Autodesk Inventor part; units mm, degrees
(part 7 of 9)
  arc A393 (-59.0073, -75.4846) -> (-59.0867, -78.0643) centre (-58.4312, -76.7934) ccw projected
  arc A394 (-58.3073, -75.2823) -> (-59.0073, -75.4846) centre (-57.9039, -77.9913) ccw projected
  arc A395 (-58.3073, -75.2823) -> (-57.8525, -74.7461) centre (-58.3858, -74.7547) ccw projected
  arc A396 (-57.8525, -74.7461) -> (-57.8729, -73.9401) centre (-101.8395, -75.4579) ccw projected
  arc A397 (-57.8729, -73.9401) -> (-58.3543, -73.4277) centre (-58.406, -73.9585) ccw projected
  arc A398 (-59.0637, -73.2611) -> (-58.3543, -73.4277) centre (-58.0887, -70.7017) ccw projected
  arc A399 (-59.2736, -70.6887) -> (-59.0637, -73.2611) centre (-58.5546, -71.9248) ccw projected
  arc A400 (-58.6006, -70.4094) -> (-59.2736, -70.6887) centre (-57.8965, -73.0561) ccw projected
  arc A401 (-58.6006, -70.4094) -> (-58.2088, -69.8256) centre (-58.7378, -69.8939) ccw projected
  arc A402 (-58.2088, -69.8256) -> (-58.3193, -69.027) centre (-101.8395, -75.4579) ccw projected
  arc A403 (-58.3193, -69.027) -> (-58.855, -68.5716) centre (-58.847, -69.105) ccw projected
  arc A404 (-59.5786, -68.4856) -> (-58.855, -68.5716) centre (-58.8963, -65.8331) ccw projected
  arc A405 (-60.0753, -65.9528) -> (-59.5786, -68.4856) centre (-59.2223, -67.1006) ccw projected
  arc A406 (-59.4378, -65.5999) -> (-60.0753, -65.9528) centre (-58.4417, -68.1512) ccw projected
  arc A407 (-59.4378, -65.5999) -> (-59.1137, -64.9759) centre (-59.6318, -65.103) ccw projected
  arc A408 (-59.1137, -64.9759) -> (-59.313, -64.1947) centre (-101.8395, -75.4579) ccw projected
  arc A409 (-59.313, -64.1947) -> (-59.8963, -63.8022) centre (-59.8286, -64.3313) ccw projected
  arc A410 (-60.625, -63.7977) -> (-59.8963, -63.8022) centre (-60.2439, -61.0855) ccw projected
  arc A411 (-61.4021, -61.3365) -> (-60.625, -63.7977) centre (-60.426, -62.3816) ccw projected
  arc A412 (-60.8081, -60.9144) -> (-61.4021, -61.3365) centre (-59.5327, -63.3381) ccw projected
  arc A413 (-60.8081, -60.9144) -> (-60.556, -60.2581) centre (-61.0566, -60.4424) ccw projected
  arc A414 (-60.556, -60.2581) -> (-60.8415, -59.5041) centre (-101.8395, -75.4579) ccw projected
  arc A415 (-60.8415, -59.5041) -> (-61.4651, -59.1793) centre (-61.3386, -59.6975) ccw projected
  arc A416 (-62.1896, -59.2564) -> (-61.4651, -59.1793) centre (-62.1147, -56.5186) ccw projected
  arc A417 (-63.2375, -56.8977) -> (-62.1896, -59.2564) centre (-62.1505, -57.827) ccw projected
  arc A418 (-62.6945, -56.4118) -> (-63.2375, -56.8977) centre (-61.1557, -58.6774) ccw projected
  arc A419 (-62.6945, -56.4118) -> (-62.5174, -55.7313) centre (-62.9942, -55.9705) ccw projected
  arc A420 (-62.5174, -55.7313) -> (-62.8855, -55.0141) centre (-101.8395, -75.4579) ccw projected
  arc A421 (-62.8855, -55.0141) -> (-63.5416, -54.7612) centre (-63.3578, -55.2619) ccw projected
  arc A422 (-64.253, -54.9189) -> (-63.5416, -54.7612) centre (-64.485, -52.19) ccw projected
  arc A423 (-65.5583, -52.6924) -> (-64.253, -54.9189) centre (-64.3741, -53.4941) ccw projected
  arc A424 (-65.0731, -52.1487) -> (-65.5583, -52.6924) centre (-63.2903, -54.2278) ccw projected
  arc A425 (-65.0731, -52.1487) -> (-64.9734, -51.4527) centre (-65.4203, -51.7438) ccw projected
  arc A426 (-64.9734, -51.4527) -> (-65.4195, -50.7811) centre (-101.8395, -75.4579) ccw projected
  arc A427 (-65.4195, -50.7811) -> (-66.0997, -50.6033) centre (-65.861, -51.0803) ccw projected
  arc A428 (-66.7889, -50.8397) -> (-66.0997, -50.6033) centre (-67.3251, -48.1539) ccw projected
  arc A429 (-68.3353, -48.7733) -> (-66.7889, -50.8397) centre (-67.0689, -49.4374) ccw projected
  arc A430 (-67.9141, -48.1787) -> (-68.3353, -48.7733) centre (-65.9097, -50.0451) ccw projected
  arc A431 (-67.9141, -48.1787) -> (-67.8929, -47.4759) centre (-68.3045, -47.8152) ccw projected
  arc A432 (-67.8929, -47.4759) -> (-68.4114, -46.8585) centre (-101.8395, -75.4579) ccw projected
  arc A433 (-68.4114, -46.8585) -> (-69.1073, -46.758) centre (-68.8167, -47.2053) ccw projected
  arc A434 (-69.7657, -47.0701) -> (-69.1073, -46.758) centre (-70.5992, -44.4612) ccw projected
  arc A435 (-71.5337, -45.1898) -> (-69.7657, -47.0701) centre (-70.2009, -45.7079) ccw projected
  arc A436 (-71.1817, -44.5518) -> (-71.5337, -45.1898) centre (-68.981, -46.1821) ccw projected
  arc A437 (-71.1817, -44.5518) -> (-71.2393, -43.8511) centre (-71.6104, -44.2343) ccw projected
  arc A438 (-71.2393, -43.8511) -> (-71.8237, -43.2956) centre (-101.8395, -75.4579) ccw projected
  arc A439 (-71.8237, -43.2956) -> (-72.5264, -43.2736) centre (-72.1876, -43.6856) ccw projected
  arc A440 (-73.1458, -43.6575) -> (-72.5264, -43.2736) centre (-74.2661, -41.1583) ccw projected
  arc A441 (-75.1132, -41.9869) -> (-73.1458, -43.6575) centre (-73.7308, -42.3525) ccw projected
  arc A442 (-74.8349, -41.3135) -> (-75.1132, -41.9869) centre (-72.4654, -42.6872) ccw projected
  arc A443 (-74.8349, -41.3135) -> (-74.9706, -40.6237) centre (-75.2964, -41.046) ccw projected
  arc A444 (-74.9706, -40.6237) -> (-75.6135, -40.1371) centre (-101.8395, -75.4579) ccw projected
  arc A445 (-75.6135, -40.1371) -> (-76.3143, -40.1939) centre (-75.9315, -40.5654) ccw projected
  arc A446 (-76.8867, -40.6447) -> (-76.3143, -40.1939) centre (-78.2798, -38.2867) ccw projected
  arc A447 (-79.0289, -39.205) -> (-76.8867, -40.6447) centre (-77.6141, -39.4135) ccw projected
  arc A448 (-78.8277, -38.5047) -> (-79.0289, -39.205) centre (-76.3193, -39.6044) ccw projected
  arc A449 (-78.8277, -38.5047) -> (-79.0397, -37.8343) centre (-79.3162, -38.2905) ccw projected
  arc A450 (-79.0397, -37.8343) -> (-79.7331, -37.4228) centre (-101.8395, -75.4579) ccw projected
  arc A451 (-79.7331, -37.4228) -> (-80.4231, -37.5577) centre (-80.0011, -37.884) ccw projected
  arc A452 (-80.9415, -38.0698) -> (-80.4231, -37.5577) centre (-82.5898, -35.8826) ccw projected
  arc A453 (-83.2313, -36.879) -> (-80.9415, -38.0698) centre (-81.8021, -36.9278) ccw projected
  arc A454 (-83.1098, -36.1605) -> (-83.2313, -36.879) centre (-80.4941, -36.9724) ccw projected
  arc A455 (-83.1098, -36.1605) -> (-83.3956, -35.5181) centre (-83.6192, -36.0024) ccw projected
  arc A456 (-83.3956, -35.5181) -> (-84.1306, -35.1868) centre (-101.8395, -75.4579) ccw projected
  line L37 (-121.8728, 32.134) -> (-90.1228, 6.734)
  line L38 (-121.8728, 6.734) -> (-90.1228, 32.134)
  circle A457 centre (-171.542, -73.2557) radius 14.2748
  circle A458 centre (-105.9978, 19.434) radius 21.4859
  circle A459 centre (-171.542, -73.2557) radius 14.3243
  line L39 (-160.3914, -82.2474) -> (-89.2724, 5.9468)
  line L40 (-124.2883, 30.7078) -> (-183.736, -65.7396)
  line L41 (-193.767, -95.4807) -> (-149.317, -95.4807)
  line L42 (-149.317, -95.4807) -> (-149.317, -51.0307)
  line L43 (-149.317, -51.0307) -> (-193.767, -51.0307)
  line L44 (-193.767, -51.0307) -> (-193.767, -95.4807)
  line L45 (-193.767, -95.4807) -> (-149.317, -51.0307) construction
  line L46 (-149.317, -95.4807) -> (-193.767, -51.0307) construction
  circle A460 centre (-171.542, -73.2557) radius 31.4309
  arc A461 (-181.9312, -110.8876) -> (-185.6678, -111.3086) centre (-183.1204, -117.1252) ccw projected
  arc A462 (-174.8852, -173.4224) -> (-181.9312, -110.8876) centre (-180.2765, -142.3655) ccw projected
  arc A463 (-178.6218, -173.8435) -> (-174.8852, -173.4224) centre (-177.4326, -167.6058) ccw projected
  arc A464 (-185.6678, -111.3086) -> (-178.6218, -173.8435) centre (-180.2765, -142.3655) ccw projected
  arc A465 (-181.7907, -98.8592) -> (-182.3406, -98.4212) centre (-182.3156, -98.954) ccw projected
  arc A466 (-182.3406, -98.4212) -> (-183.1456, -98.4664) centre (-180.2765, -142.3655) ccw projected
  arc A467 (-183.1456, -98.4664) -> (-183.643, -98.9632) centre (-183.1108, -98.9986) ccw projected
  arc A468 (-183.7876, -99.6774) -> (-183.643, -98.9632) centre (-186.3758, -98.7816) ccw projected
  arc A469 (-186.3524, -99.9664) -> (-183.7876, -99.6774) centre (-185.139, -99.2097) ccw projected
  arc A470 (-186.6523, -99.3023) -> (-186.3524, -99.9664) centre (-184.0285, -98.5171) ccw projected
  arc A471 (-186.6523, -99.3023) -> (-187.2478, -98.9286) centre (-187.1633, -99.4552) ccw projected
  arc A472 (-187.2478, -98.9286) -> (-188.0427, -99.0636) centre (-180.2765, -142.3655) ccw projected
  arc A473 (-188.0427, -99.0636) -> (-188.4814, -99.6131) centre (-187.9485, -99.5887) ccw projected
  arc A474 (-188.5451, -100.3389) -> (-188.4814, -99.6131) centre (-191.2173, -99.7385) ccw projected
  arc A475 (-191.0614, -100.9133) -> (-188.5451, -100.3389) centre (-189.9403, -100.0254) ccw projected
  arc A476 (-191.4338, -100.2869) -> (-191.0614, -100.9133) centre (-188.9143, -99.2129) ccw projected
  arc A477 (-191.4338, -100.2869) -> (-192.0674, -99.9822) centre (-191.9244, -100.4961) ccw projected
  arc A478 (-192.0674, -99.9822) -> (-192.8421, -100.2054) centre (-180.2765, -142.3655) ccw projected
  arc A479 (-192.8421, -100.2054) -> (-193.2165, -100.8006) centre (-192.6898, -100.7166) ccw projected
  arc A480 (-193.1986, -101.529) -> (-193.2165, -100.8006) centre (-195.9212, -101.2315) ccw projected
  arc A481 (-195.6348, -102.3814) -> (-193.1986, -101.529) centre (-194.6202, -101.3737) ccw projected
  arc A482 (-196.0749, -101.8007) -> (-195.6348, -102.3814) centre (-193.6916, -100.4513) ccw projected
  arc A483 (-196.0749, -101.8007) -> (-196.7387, -101.5689) centre (-196.5391, -102.0636) ccw projected
  arc A484 (-196.7387, -101.5689) -> (-197.4835, -101.8774) centre (-180.2765, -142.3655) ccw projected
  arc A485 (-197.4835, -101.8774) -> (-197.789, -102.5107) centre (-197.2749, -102.3683) ccw projected
  arc A486 (-197.6896, -103.2326) -> (-197.789, -102.5107) centre (-200.4284, -103.2418) ccw projected
  arc A487 (-200.015, -104.3524) -> (-197.6896, -103.2326) centre (-199.1196, -103.2374) ccw projected
  arc A488 (-200.5174, -103.8247) -> (-200.015, -104.3524) centre (-198.3001, -102.2169) ccw projected
  arc A489 (-200.5174, -103.8247) -> (-201.2029, -103.6686) centre (-200.9492, -104.1378) ccw projected
  arc A490 (-201.2029, -103.6686) -> (-201.9086, -104.0586) centre (-180.2765, -142.3655) ccw projected
  arc A491 (-201.9086, -104.0586) -> (-202.1412, -104.7221) centre (-201.6463, -104.5231) ccw projected
  arc A492 (-201.9616, -105.4283) -> (-202.1412, -104.7221) centre (-204.6822, -105.7441) ccw projected
  arc A493 (-204.147, -106.8014) -> (-201.9616, -105.4283) centre (-203.3821, -105.5932) ccw projected
  arc A494 (-204.7053, -106.3333) -> (-204.147, -106.8014) centre (-202.682, -104.4874) ccw projected
  arc A495 (-204.7053, -106.3333) -> (-205.404, -106.2549) centre (-205.0994, -106.6928) ccw projected
  arc A496 (-205.404, -106.2549) -> (-206.0616, -106.7215) centre (-180.2765, -142.3655) ccw projected
  arc A497 (-206.0616, -106.7215) -> (-206.2184, -107.4069) centre (-205.7489, -107.1537) ccw projected
  arc A498 (-205.9609, -108.0885) -> (-206.2184, -107.4069) centre (-208.629, -108.707) ccw projected
  arc A499 (-207.9788, -109.6977) -> (-205.9609, -108.0885) centre (-207.354, -108.4114) ccw projected
  arc A500 (-208.5861, -109.295) -> (-207.9788, -109.6977) centre (-206.7821, -107.2342) ccw projected
  arc A501 (-208.5861, -109.295) -> (-209.2891, -109.2954) centre (-208.9374, -109.6964) ccw projected
  arc A502 (-209.2891, -109.2954) -> (-209.8903, -109.8326) centre (-180.2765, -142.3655) ccw projected
  arc A503 (-209.8903, -109.8326) -> (-209.9694, -110.5312) centre (-209.5312, -110.2271) ccw projected
  arc A504 (-209.6372, -111.1798) -> (-209.9694, -110.5312) centre (-212.2193, -112.0931) ccw projected
  arc A505 (-211.4623, -113.0048) -> (-209.6372, -111.1798) centre (-210.9854, -111.6566) ccw projected
  arc A506 (-212.1108, -112.6726) -> (-211.4623, -113.0048) centre (-210.5489, -110.4227) ccw projected
  arc A507 (-212.1108, -112.6726) -> (-212.8094, -112.7517) centre (-212.4149, -113.1108) ccw projected
  arc A508 (-212.8094, -112.7517) -> (-213.3466, -113.3529) centre (-180.2765, -142.3655) ccw projected
  arc A509 (-213.3466, -113.3529) -> (-213.347, -114.056) centre (-212.9457, -113.7046) ccw projected
  arc A510 (-212.9443, -114.6632) -> (-213.347, -114.056) centre (-215.4079, -115.8599) ccw projected
  arc A511 (-214.5535, -116.6811) -> (-212.9443, -114.6632) centre (-214.2306, -115.288) ccw projected
  arc A512 (-215.2352, -116.4236) -> (-214.5535, -116.6811) centre (-213.9351, -114.013) ccw projected
  arc A513 (-215.2352, -116.4236) -> (-215.9205, -116.5804) centre (-215.4884, -116.8931) ccw projected
  arc A514 (-215.9205, -116.5804) -> (-216.3871, -117.238) centre (-180.2765, -142.3655) ccw projected
  arc A515 (-216.3871, -117.238) -> (-216.3087, -117.9367) centre (-215.9492, -117.5426) ccw projected
  arc A516 (-215.8406, -118.495) -> (-216.3087, -117.9367) centre (-218.1547, -119.96) ccw projected
  arc A517 (-217.2137, -120.6804) -> (-215.8406, -118.495) centre (-217.0488, -119.2599) ccw projected
  arc A518 (-217.9199, -120.5008) -> (-217.2137, -120.6804) centre (-216.8979, -117.9599) ccw projected
  arc A519 (-217.9199, -120.5008) -> (-218.5834, -120.7334) centre (-218.119, -120.9957) ccw projected
  arc A520 (-218.5834, -120.7334) -> (-218.9734, -121.4391) centre (-180.2765, -142.3655) ccw projected
  arc A521 (-218.9734, -121.4391) -> (-218.8173, -122.1246) centre (-218.5042, -121.6928) ccw projected
  arc A522 (-218.2896, -122.627) -> (-218.8173, -122.1246) centre (-220.4251, -124.3419) ccw projected
  arc A523 (-219.4094, -124.9524) -> (-218.2896, -122.627) centre (-219.4046, -123.5224) ccw projected
  arc A524 (-220.1313, -124.8531) -> (-219.4094, -124.9524) centre (-219.4002, -122.2136) ccw projected
  arc A525 (-220.1313, -124.8531) -> (-220.7646, -125.1585) centre (-220.2737, -125.3671) ccw projected
  arc A526 (-220.7646, -125.1585) -> (-221.0731, -125.9033) centre (-180.2765, -142.3655) ccw projected
  arc A527 (-221.0731, -125.9033) -> (-220.8413, -126.5671) centre (-220.5785, -126.1029) ccw projected
  arc A528 (-220.2606, -127.0073) -> (-220.8413, -126.5671) centre (-222.1907, -128.9504) ccw projected
  arc A529 (-221.113, -129.4434) -> (-220.2606, -127.0073) centre (-221.2683, -128.0218) ccw projected
  arc A530 (-221.8415, -129.4255) -> (-221.113, -129.4434) centre (-221.4105, -126.7208) ccw projected
  arc A531 (-221.8415, -129.4255) -> (-222.4366, -129.7999) centre (-221.9254, -129.9522) ccw projected
  arc A532 (-222.4366, -129.7999) -> (-222.6598, -130.5746) centre (-180.2765, -142.3655) ccw projected
  arc A533 (-222.6598, -130.5746) -> (-222.3551, -131.2083) centre (-222.1459, -130.7176) ccw projected
  arc A534 (-221.7287, -131.5806) -> (-222.3551, -131.2083) centre (-223.4291, -133.7277) ccw projected
  arc A535 (-222.3031, -134.0969) -> (-221.7287, -131.5806) centre (-222.6166, -132.7017) ccw projected
  arc A536 (-223.0289, -134.1607) -> (-222.3031, -134.0969) centre (-222.9035, -131.4247) ccw projected
  arc A537 (-223.0289, -134.1607) -> (-223.5784, -134.5993) centre (-223.0534, -134.6935) ccw projected
  arc A538 (-223.5784, -134.5993) -> (-223.7134, -135.3942) centre (-180.2765, -142.3655) ccw projected
  arc A539 (-223.7134, -135.3942) -> (-223.3397, -135.9897) centre (-223.1868, -135.4787) ccw projected
  arc A540 (-222.6756, -136.2896) -> (-223.3397, -135.9897) centre (-224.1249, -138.6136) ccw projected
  arc A541 (-222.9646, -138.8544) -> (-222.6756, -136.2896) centre (-223.4324, -137.503) ccw projected
  arc A542 (-223.6788, -138.999) -> (-222.9646, -138.8544) centre (-223.8604, -136.2662) ccw projected
  arc A543 (-223.6788, -138.999) -> (-224.1756, -139.4964) centre (-223.6434, -139.5312) ccw projected
  arc A544 (-224.1756, -139.4964) -> (-224.2209, -140.3014) centre (-180.2765, -142.3655) ccw projected
  arc A545 (-224.2209, -140.3014) -> (-223.7828, -140.8513) centre (-223.688, -140.3264) ccw projected
  arc A546 (-223.0893, -141.075) -> (-223.7828, -140.8513) centre (-224.2693, -143.5466) ccw projected
  arc A547 (-223.0893, -143.656) -> (-223.0893, -141.075) centre (-223.7054, -142.3655) ccw projected
  arc A548 (-223.7828, -143.8797) -> (-223.0893, -143.656) centre (-224.2693, -141.1844) ccw projected
  arc A549 (-223.7828, -143.8797) -> (-224.2209, -144.4296) centre (-223.688, -144.4046) ccw projected
  arc A550 (-224.2209, -144.4296) -> (-224.1756, -145.2346) centre (-180.2765, -142.3655) ccw projected
  arc A551 (-224.1756, -145.2346) -> (-223.6788, -145.732) centre (-223.6434, -145.1998) ccw projected
  arc A552 (-222.9646, -145.8766) -> (-223.6788, -145.732) centre (-223.8604, -148.4648) ccw projected
  arc A553 (-222.6756, -148.4414) -> (-222.9646, -145.8766) centre (-223.4324, -147.228) ccw projected
  arc A554 (-223.3397, -148.7413) -> (-222.6756, -148.4414) centre (-224.1249, -146.1175) ccw projected
  arc A555 (-223.3397, -148.7413) -> (-223.7134, -149.3368) centre (-223.1868, -149.2523) ccw projected
  arc A556 (-223.7134, -149.3368) -> (-223.5784, -150.1317) centre (-180.2765, -142.3655) ccw projected
  arc A557 (-223.5784, -150.1317) -> (-223.0289, -150.5704) centre (-223.0534, -150.0375) ccw projected
  arc A558 (-222.3031, -150.6341) -> (-223.0289, -150.5704) centre (-222.9035, -153.3063) ccw projected
  arc A559 (-221.7287, -153.1504) -> (-222.3031, -150.6341) centre (-222.6166, -152.0294) ccw projected
  arc A560 (-222.3551, -153.5228) -> (-221.7287, -153.1504) centre (-223.4291, -151.0033) ccw projected
  arc A561 (-222.3551, -153.5228) -> (-222.6598, -154.1564) centre (-222.1459, -154.0134) ccw projected
  arc A562 (-222.6598, -154.1564) -> (-222.4366, -154.9311) centre (-180.2765, -142.3655) ccw projected
  arc A563 (-222.4366, -154.9311) -> (-221.8415, -155.3055) centre (-221.9254, -154.7788) ccw projected
  arc A564 (-221.113, -155.2876) -> (-221.8415, -155.3055) centre (-221.4105, -158.0102) ccw projected
  arc A565 (-220.2606, -157.7238) -> (-221.113, -155.2876) centre (-221.2683, -156.7092) ccw projected
  arc A566 (-220.8413, -158.1639) -> (-220.2606, -157.7238) centre (-222.1907, -155.7806) ccw projected
  arc A567 (-220.8413, -158.1639) -> (-221.0731, -158.8277) centre (-220.5785, -158.6281) ccw projected
  arc A568 (-221.0731, -158.8277) -> (-220.7646, -159.5726) centre (-180.2765, -142.3655) ccw projected
  arc A569 (-220.7646, -159.5726) -> (-220.1313, -159.878) centre (-220.2737, -159.3639) ccw projected
  arc A570 (-219.4094, -159.7786) -> (-220.1313, -159.878) centre (-219.4002, -162.5174) ccw projected
  arc A571 (-218.2896, -162.104) -> (-219.4094, -159.7786) centre (-219.4046, -161.2086) ccw projected
  arc A572 (-218.8173, -162.6064) -> (-218.2896, -162.104) centre (-220.4251, -160.3891) ccw projected
  arc A573 (-218.8173, -162.6064) -> (-218.9734, -163.2919) centre (-218.5042, -163.0382) ccw projected
  arc A574 (-218.9734, -163.2919) -> (-218.5834, -163.9976) centre (-180.2765, -142.3655) ccw projected
  arc A575 (-218.5834, -163.9976) -> (-217.9199, -164.2302) centre (-218.119, -163.7353) ccw projected
  arc A576 (-217.2137, -164.0506) -> (-217.9199, -164.2302) centre (-216.8979, -166.7712) ccw projected
  arc A577 (-215.8406, -166.236) -> (-217.2137, -164.0506) centre (-217.0488, -165.4711) ccw projected
  arc A578 (-216.3087, -166.7943) -> (-215.8406, -166.236) centre (-218.1547, -164.771) ccw projected
  arc A579 (-216.3087, -166.7943) -> (-216.3871, -167.493) centre (-215.9492, -167.1884) ccw projected
  arc A580 (-216.3871, -167.493) -> (-215.9205, -168.1506) centre (-180.2765, -142.3655) ccw projected
  arc A581 (-215.9205, -168.1506) -> (-215.2352, -168.3074) centre (-215.4884, -167.8379) ccw projected
  arc A582 (-214.5535, -168.0499) -> (-215.2352, -168.3074) centre (-213.9351, -170.718) ccw projected
  arc A583 (-212.9443, -170.0678) -> (-214.5535, -168.0499) centre (-214.2306, -169.443) ccw projected
  arc A584 (-213.347, -170.6751) -> (-212.9443, -170.0678) centre (-215.4079, -168.8712) ccw projected
  arc A585 (-213.347, -170.6751) -> (-213.3466, -171.3781) centre (-212.9457, -171.0264) ccw projected
  arc A586 (-213.3466, -171.3781) -> (-212.8094, -171.9793) centre (-180.2765, -142.3655) ccw projected
  arc A587 (-212.8094, -171.9793) -> (-212.1108, -172.0584) centre (-212.4149, -171.6203) ccw projected
  arc A588 (-211.4623, -171.7262) -> (-212.1108, -172.0584) centre (-210.5489, -174.3083) ccw projected
  arc A589 (-209.6372, -173.5513) -> (-211.4623, -171.7262) centre (-210.9854, -173.0744) ccw projected
  arc A590 (-209.9694, -174.1998) -> (-209.6372, -173.5513) centre (-212.2193, -172.638) ccw projected
  arc A591 (-209.9694, -174.1998) -> (-209.8903, -174.8984) centre (-209.5312, -174.504) ccw projected
  arc A592 (-209.8903, -174.8984) -> (-209.2891, -175.4356) centre (-180.2765, -142.3655) ccw projected
  arc A593 (-209.2891, -175.4356) -> (-208.5861, -175.436) centre (-208.9374, -175.0347) ccw projected
  arc A594 (-207.9788, -175.0333) -> (-208.5861, -175.436) centre (-206.7821, -177.4969) ccw projected
  arc A595 (-205.9609, -176.6425) -> (-207.9788, -175.0333) centre (-207.354, -176.3196) ccw projected
  arc A596 (-206.2184, -177.3242) -> (-205.9609, -176.6425) centre (-208.629, -176.0241) ccw projected
  arc A597 (-206.2184, -177.3242) -> (-206.0616, -178.0095) centre (-205.7489, -177.5774) ccw projected
  arc A598 (-206.0616, -178.0095) -> (-205.404, -178.4761) centre (-180.2765, -142.3655) ccw projected
  arc A599 (-205.404, -178.4761) -> (-204.7053, -178.3978) centre (-205.0994, -178.0383) ccw projected
  arc A600 (-204.147, -177.9296) -> (-204.7053, -178.3978) centre (-202.682, -180.2437) ccw projected
  arc A601 (-201.9616, -179.3027) -> (-204.147, -177.9296) centre (-203.3821, -179.1378) ccw projected
  arc A602 (-202.1412, -180.0089) -> (-201.9616, -179.3027) centre (-204.6822, -178.9869) ccw projected
  arc A603 (-202.1412, -180.0089) -> (-201.9086, -180.6724) centre (-201.6463, -180.208) ccw projected
  arc A604 (-201.9086, -180.6724) -> (-201.2029, -181.0624) centre (-180.2765, -142.3655) ccw projected
  arc A605 (-201.2029, -181.0624) -> (-200.5174, -180.9064) centre (-200.9492, -180.5932) ccw projected
  arc A606 (-200.015, -180.3786) -> (-200.5174, -180.9064) centre (-198.3001, -182.5141) ccw projected
  arc A607 (-197.6896, -181.4984) -> (-200.015, -180.3786) centre (-199.1196, -181.4936) ccw projected
  arc A608 (-197.789, -182.2203) -> (-197.6896, -181.4984) centre (-200.4284, -181.4892) ccw projected
  arc A609 (-197.789, -182.2203) -> (-197.4835, -182.8536) centre (-197.2749, -182.3627) ccw projected
  arc A610 (-197.4835, -182.8536) -> (-196.7387, -183.1621) centre (-180.2765, -142.3655) ccw projected
  arc A611 (-196.7387, -183.1621) -> (-196.0749, -182.9303) centre (-196.5391, -182.6675) ccw projected
  arc A612 (-195.6348, -182.3496) -> (-196.0749, -182.9303) centre (-193.6916, -184.2797) ccw projected
  arc A613 (-193.1986, -183.202) -> (-195.6348, -182.3496) centre (-194.6202, -183.3573) ccw projected
  arc A614 (-193.2165, -183.9305) -> (-193.1986, -183.202) centre (-195.9212, -183.4995) ccw projected
  arc A615 (-193.2165, -183.9305) -> (-192.8421, -184.5256) centre (-192.6898, -184.0144) ccw projected
  arc A616 (-192.8421, -184.5256) -> (-192.0674, -184.7488) centre (-180.2765, -142.3655) ccw projected
  arc A617 (-192.0674, -184.7488) -> (-191.4338, -184.4441) centre (-191.9244, -184.2349) ccw projected
  arc A618 (-191.0614, -183.8178) -> (-191.4338, -184.4441) centre (-188.9143, -185.5181) ccw projected
  arc A619 (-188.5451, -184.3921) -> (-191.0614, -183.8178) centre (-189.9403, -184.7056) ccw projected
  arc A620 (-188.4814, -185.1179) -> (-188.5451, -184.3921) centre (-191.2173, -184.9925) ccw projected
  arc A621 (-188.4814, -185.1179) -> (-188.0427, -185.6674) centre (-187.9485, -185.1424) ccw projected
  arc A622 (-188.0427, -185.6674) -> (-187.2478, -185.8024) centre (-180.2765, -142.3655) ccw projected
  arc A623 (-187.2478, -185.8024) -> (-186.6523, -185.4287) centre (-187.1633, -185.2758) ccw projected
  arc A624 (-186.3524, -184.7646) -> (-186.6523, -185.4287) centre (-184.0285, -186.2139) ccw projected
  arc A625 (-183.7876, -185.0536) -> (-186.3524, -184.7646) centre (-185.139, -185.5214) ccw projected
  arc A626 (-183.643, -185.7678) -> (-183.7876, -185.0536) centre (-186.3758, -185.9495) ccw projected
  arc A627 (-183.643, -185.7678) -> (-183.1456, -186.2647) centre (-183.1108, -185.7324) ccw projected
  arc A628 (-183.1456, -186.2647) -> (-182.3406, -186.3099) centre (-180.2765, -142.3655) ccw projected
  arc A629 (-182.3406, -186.3099) -> (-181.7907, -185.8718) centre (-182.3156, -185.777) ccw projected
  arc A630 (-181.567, -185.1783) -> (-181.7907, -185.8718) centre (-179.0954, -186.3583) ccw projected
  arc A631 (-178.986, -185.1783) -> (-181.567, -185.1783) centre (-180.2765, -185.7944) ccw projected
  arc A632 (-178.7623, -185.8718) -> (-178.986, -185.1783) centre (-181.4576, -186.3583) ccw projected
  arc A633 (-178.7623, -185.8718) -> (-178.2124, -186.3099) centre (-178.2374, -185.777) ccw projected
  arc A634 (-178.2124, -186.3099) -> (-177.4074, -186.2647) centre (-180.2765, -142.3655) ccw projected
  arc A635 (-177.4074, -186.2647) -> (-176.91, -185.7678) centre (-177.4422, -185.7324) ccw projected
  arc A636 (-176.7654, -185.0536) -> (-176.91, -185.7678) centre (-174.1772, -185.9495) ccw projected
  arc A637 (-174.2006, -184.7646) -> (-176.7654, -185.0536) centre (-175.414, -185.5214) ccw projected
  arc A638 (-173.9007, -185.4287) -> (-174.2006, -184.7646) centre (-176.5245, -186.2139) ccw projected
  arc A639 (-173.9007, -185.4287) -> (-173.3052, -185.8024) centre (-173.3897, -185.2758) ccw projected
  arc A640 (-173.3052, -185.8024) -> (-172.5103, -185.6674) centre (-180.2765, -142.3655) ccw projected
  arc A641 (-172.5103, -185.6674) -> (-172.0716, -185.1179) centre (-172.6045, -185.1424) ccw projected
  arc A642 (-172.0079, -184.3921) -> (-172.0716, -185.1179) centre (-169.3357, -184.9925) ccw projected
  arc A643 (-169.4916, -183.8178) -> (-172.0079, -184.3921) centre (-170.6127, -184.7056) ccw projected
  arc A644 (-169.1192, -184.4441) -> (-169.4916, -183.8178) centre (-171.6387, -185.5181) ccw projected
  arc A645 (-169.1192, -184.4441) -> (-168.4856, -184.7488) centre (-168.6286, -184.2349) ccw projected
  arc A646 (-168.4856, -184.7488) -> (-167.7109, -184.5256) centre (-180.2765, -142.3655) ccw projected
  arc A647 (-167.7109, -184.5256) -> (-167.3365, -183.9305) centre (-167.8632, -184.0144) ccw projected
  arc A648 (-167.3544, -183.202) -> (-167.3365, -183.9305) centre (-164.6318, -183.4995) ccw projected
  arc A649 (-164.9183, -182.3496) -> (-167.3544, -183.202) centre (-165.9328, -183.3573) ccw projected
  arc A650 (-164.4781, -182.9303) -> (-164.9183, -182.3496) centre (-166.8614, -184.2797) ccw projected
  arc A651 (-164.4781, -182.9303) -> (-163.8143, -183.1621) centre (-164.0139, -182.6675) ccw projected
  arc A652 (-163.8143, -183.1621) -> (-163.0695, -182.8536) centre (-180.2765, -142.3655) ccw projected
  arc A653 (-163.0695, -182.8536) -> (-162.764, -182.2203) centre (-163.2781, -182.3627) ccw projected
  arc A654 (-162.8634, -181.4984) -> (-162.764, -182.2203) centre (-160.1246, -181.4892) ccw projected
  arc A655 (-160.538, -180.3786) -> (-162.8634, -181.4984) centre (-161.4334, -181.4936) ccw projected
  arc A656 (-160.0356, -180.9064) -> (-160.538, -180.3786) centre (-162.2529, -182.5141) ccw projected
  arc A657 (-160.0356, -180.9064) -> (-159.3501, -181.0624) centre (-159.6038, -180.5932) ccw projected
  arc A658 (-159.3501, -181.0624) -> (-158.6444, -180.6724) centre (-180.2765, -142.3655) ccw projected
  arc A659 (-158.6444, -180.6724) -> (-158.4118, -180.0089) centre (-158.9067, -180.208) ccw projected
  arc A660 (-158.5914, -179.3027) -> (-158.4118, -180.0089) centre (-155.8709, -178.9869) ccw projected
  arc A661 (-156.406, -177.9296) -> (-158.5914, -179.3027) centre (-157.1709, -179.1378) ccw projected
  arc A662 (-155.8477, -178.3978) -> (-156.406, -177.9296) centre (-157.871, -180.2437) ccw projected
  arc A663 (-155.8477, -178.3978) -> (-155.149, -178.4761) centre (-155.4536, -178.0383) ccw projected
  arc A664 (-155.149, -178.4761) -> (-154.4914, -178.0095) centre (-180.2765, -142.3655) ccw projected
  arc A665 (-154.4914, -178.0095) -> (-154.3346, -177.3242) centre (-154.8041, -177.5774) ccw projected
  arc A666 (-154.5921, -176.6425) -> (-154.3346, -177.3242) centre (-151.924, -176.0241) ccw projected
  arc A667 (-152.5742, -175.0333) -> (-154.5921, -176.6425) centre (-153.199, -176.3196) ccw projected
  arc A668 (-151.967, -175.436) -> (-152.5742, -175.0333) centre (-153.7709, -177.4969) ccw projected
  arc A669 (-151.967, -175.436) -> (-151.2639, -175.4356) centre (-151.6156, -175.0347) ccw projected
  arc A670 (-151.2639, -175.4356) -> (-150.6627, -174.8984) centre (-180.2765, -142.3655) ccw projected
  arc A671 (-150.6627, -174.8984) -> (-150.5836, -174.1998) centre (-151.0218, -174.504) ccw projected
  arc A672 (-150.9158, -173.5513) -> (-150.5836, -174.1998) centre (-148.3337, -172.638) ccw projected
  arc A673 (-149.0908, -171.7262) -> (-150.9158, -173.5513) centre (-149.5676, -173.0744) ccw projected
  arc A674 (-148.4422, -172.0584) -> (-149.0908, -171.7262) centre (-150.0041, -174.3083) ccw projected
  arc A675 (-148.4422, -172.0584) -> (-147.7436, -171.9793) centre (-148.1381, -171.6203) ccw projected
  arc A676 (-147.7436, -171.9793) -> (-147.2064, -171.3781) centre (-180.2765, -142.3655) ccw projected
  arc A677 (-147.2064, -171.3781) -> (-147.206, -170.6751) centre (-147.6073, -171.0264) ccw projected
  arc A678 (-147.6087, -170.0678) -> (-147.206, -170.6751) centre (-145.1451, -168.8712) ccw projected
  arc A679 (-145.9995, -168.0499) -> (-147.6087, -170.0678) centre (-146.3224, -169.443) ccw projected
  arc A680 (-145.3179, -168.3074) -> (-145.9995, -168.0499) centre (-146.618, -170.718) ccw projected
  arc A681 (-145.3179, -168.3074) -> (-144.6325, -168.1506) centre (-145.0647, -167.8379) ccw projected
  arc A682 (-144.6325, -168.1506) -> (-144.1659, -167.493) centre (-180.2765, -142.3655) ccw projected
  arc A683 (-144.1659, -167.493) -> (-144.2443, -166.7943) centre (-144.6038, -167.1884) ccw projected
  arc A684 (-144.7124, -166.236) -> (-144.2443, -166.7943) centre (-142.3984, -164.771) ccw projected
  arc A685 (-143.3393, -164.0506) -> (-144.7124, -166.236) centre (-143.5042, -165.4711) ccw projected
  arc A686 (-142.6331, -164.2302) -> (-143.3393, -164.0506) centre (-143.6551, -166.7712) ccw projected
  arc A687 (-142.6331, -164.2302) -> (-141.9696, -163.9976) centre (-142.434, -163.7353) ccw projected
  arc A688 (-141.9696, -163.9976) -> (-141.5796, -163.2919) centre (-180.2765, -142.3655) ccw projected
  arc A689 (-141.5796, -163.2919) -> (-141.7357, -162.6064) centre (-142.0488, -163.0382) ccw projected
  arc A690 (-142.2634, -162.104) -> (-141.7357, -162.6064) centre (-140.1279, -160.3891) ccw projected
  arc A691 (-141.1436, -159.7786) -> (-142.2634, -162.104) centre (-141.1484, -161.2086) ccw projected
  arc A692 (-140.4217, -159.878) -> (-141.1436, -159.7786) centre (-141.1528, -162.5174) ccw projected
  arc A693 (-140.4217, -159.878) -> (-139.7884, -159.5726) centre (-140.2793, -159.3639) ccw projected
  arc A694 (-139.7884, -159.5726) -> (-139.4799, -158.8277) centre (-180.2765, -142.3655) ccw projected
  arc A695 (-139.4799, -158.8277) -> (-139.7117, -158.1639) centre (-139.9745, -158.6281) ccw projected
  arc A696 (-140.2924, -157.7238) -> (-139.7117, -158.1639) centre (-138.3623, -155.7806) ccw projected
  arc A697 (-139.44, -155.2876) -> (-140.2924, -157.7238) centre (-139.2847, -156.7092) ccw projected
  arc A698 (-138.7115, -155.3055) -> (-139.44, -155.2876) centre (-139.1425, -158.0102) ccw projected
  arc A699 (-138.7115, -155.3055) -> (-138.1164, -154.9311) centre (-138.6276, -154.7788) ccw projected
  arc A700 (-138.1164, -154.9311) -> (-137.8932, -154.1564) centre (-180.2765, -142.3655) ccw projected
  arc A701 (-137.8932, -154.1564) -> (-138.1979, -153.5228) centre (-138.4071, -154.0134) ccw projected
  arc A702 (-138.8243, -153.1504) -> (-138.1979, -153.5228) centre (-137.1239, -151.0033) ccw projected
  arc A703 (-138.2499, -150.6341) -> (-138.8243, -153.1504) centre (-137.9364, -152.0294) ccw projected
  arc A704 (-137.5241, -150.5704) -> (-138.2499, -150.6341) centre (-137.6495, -153.3063) ccw projected
  arc A705 (-137.5241, -150.5704) -> (-136.9746, -150.1317) centre (-137.4996, -150.0375) ccw projected
  arc A706 (-136.9746, -150.1317) -> (-136.8396, -149.3368) centre (-180.2765, -142.3655) ccw projected
  arc A707 (-136.8396, -149.3368) -> (-137.2133, -148.7413) centre (-137.3662, -149.2523) ccw projected
  arc A708 (-137.8774, -148.4414) -> (-137.2133, -148.7413) centre (-136.4281, -146.1175) ccw projected
  arc A709 (-137.5884, -145.8766) -> (-137.8774, -148.4414) centre (-137.1207, -147.228) ccw projected
  arc A710 (-136.8742, -145.732) -> (-137.5884, -145.8766) centre (-136.6926, -148.4648) ccw projected
  arc A711 (-136.8742, -145.732) -> (-136.3774, -145.2346) centre (-136.9096, -145.1998) ccw projected
  arc A712 (-136.3774, -145.2346) -> (-136.3322, -144.4296) centre (-180.2765, -142.3655) ccw projected
  arc A713 (-136.3322, -144.4296) -> (-136.7702, -143.8797) centre (-136.865, -144.4046) ccw projected
  arc A714 (-137.4637, -143.656) -> (-136.7702, -143.8797) centre (-136.2837, -141.1844) ccw projected
  arc A715 (-137.4637, -141.075) -> (-137.4637, -143.656) centre (-136.8476, -142.3655) ccw projected
  arc A716 (-136.7702, -140.8513) -> (-137.4637, -141.075) centre (-136.2837, -143.5466) ccw projected
  arc A717 (-136.7702, -140.8513) -> (-136.3322, -140.3014) centre (-136.865, -140.3264) ccw projected
  arc A718 (-136.3322, -140.3014) -> (-136.3774, -139.4964) centre (-180.2765, -142.3655) ccw projected
  arc A719 (-136.3774, -139.4964) -> (-136.8742, -138.999) centre (-136.9096, -139.5312) ccw projected
  arc A720 (-137.5884, -138.8544) -> (-136.8742, -138.999) centre (-136.6926, -136.2662) ccw projected
  arc A721 (-137.8774, -136.2896) -> (-137.5884, -138.8544) centre (-137.1207, -137.503) ccw projected
  arc A722 (-137.2133, -135.9897) -> (-137.8774, -136.2896) centre (-136.4281, -138.6136) ccw projected
  arc A723 (-137.2133, -135.9897) -> (-136.8396, -135.3942) centre (-137.3662, -135.4787) ccw projected
  arc A724 (-136.8396, -135.3942) -> (-136.9746, -134.5993) centre (-180.2765, -142.3655) ccw projected
  arc A725 (-136.9746, -134.5993) -> (-137.5241, -134.1607) centre (-137.4996, -134.6935) ccw projected
  arc A726 (-138.2499, -134.0969) -> (-137.5241, -134.1607) centre (-137.6495, -131.4247) ccw projected
  arc A727 (-138.8243, -131.5806) -> (-138.2499, -134.0969) centre (-137.9364, -132.7017) ccw projected
  arc A728 (-138.1979, -131.2083) -> (-138.8243, -131.5806) centre (-137.1239, -133.7277) ccw projected
  arc A729 (-138.1979, -131.2083) -> (-137.8932, -130.5746) centre (-138.4071, -130.7176) ccw projected
  arc A730 (-137.8932, -130.5746) -> (-138.1164, -129.7999) centre (-180.2765, -142.3655) ccw projected
  arc A731 (-138.1164, -129.7999) -> (-138.7115, -129.4255) centre (-138.6276, -129.9522) ccw projected
  arc A732 (-139.44, -129.4434) -> (-138.7115, -129.4255) centre (-139.1425, -126.7208) ccw projected
  arc A733 (-140.2924, -127.0073) -> (-139.44, -129.4434) centre (-139.2847, -128.0218) ccw projected
  arc A734 (-139.7117, -126.5671) -> (-140.2924, -127.0073) centre (-138.3623, -128.9504) ccw projected
  arc A735 (-139.7117, -126.5671) -> (-139.4799, -125.9033) centre (-139.9745, -126.1029) ccw projected
  arc A736 (-139.4799, -125.9033) -> (-139.7884, -125.1585) centre (-180.2765, -142.3655) ccw projected
  arc A737 (-139.7884, -125.1585) -> (-140.4217, -124.8531) centre (-140.2793, -125.3671) ccw projected
  arc A738 (-141.1436, -124.9524) -> (-140.4217, -124.8531) centre (-141.1528, -122.2136) ccw projected
  arc A739 (-142.2634, -122.627) -> (-141.1436, -124.9524) centre (-141.1484, -123.5224) ccw projected
  arc A740 (-141.7357, -122.1246) -> (-142.2634, -122.627) centre (-140.1279, -124.3419) ccw projected
  arc A741 (-141.7357, -122.1246) -> (-141.5796, -121.4391) centre (-142.0488, -121.6928) ccw projected
  arc A742 (-141.5796, -121.4391) -> (-141.9696, -120.7334) centre (-180.2765, -142.3655) ccw projected
  arc A743 (-141.9696, -120.7334) -> (-142.6331, -120.5008) centre (-142.434, -120.9957) ccw projected
  arc A744 (-143.3393, -120.6804) -> (-142.6331, -120.5008) centre (-143.6551, -117.9599) ccw projected
  arc A745 (-144.7124, -118.495) -> (-143.3393, -120.6804) centre (-143.5042, -119.2599) ccw projected
  arc A746 (-144.2443, -117.9367) -> (-144.7124, -118.495) centre (-142.3984, -119.96) ccw projected
  arc A747 (-144.2443, -117.9367) -> (-144.1659, -117.238) centre (-144.6038, -117.5426) ccw projected
  arc A748 (-144.1659, -117.238) -> (-144.6325, -116.5804) centre (-180.2765, -142.3655) ccw projected
  arc A749 (-144.6325, -116.5804) -> (-145.3179, -116.4236) centre (-145.0647, -116.8931) ccw projected
  arc A750 (-145.9995, -116.6811) -> (-145.3179, -116.4236) centre (-146.618, -114.013) ccw projected
  arc A751 (-147.6087, -114.6632) -> (-145.9995, -116.6811) centre (-146.3224, -115.288) ccw projected
  arc A752 (-147.206, -114.056) -> (-147.6087, -114.6632) centre (-145.1451, -115.8599) ccw projected
  arc A753 (-147.206, -114.056) -> (-147.2064, -113.3529) centre (-147.6073, -113.7046) ccw projected
  arc A754 (-147.2064, -113.3529) -> (-147.7436, -112.7517) centre (-180.2765, -142.3655) ccw projected
  arc A755 (-147.7436, -112.7517) -> (-148.4422, -112.6726) centre (-148.1381, -113.1108) ccw projected
  arc A756 (-149.0908, -113.0048) -> (-148.4422, -112.6726) centre (-150.0041, -110.4227) ccw projected
  arc A757 (-150.9158, -111.1798) -> (-149.0908, -113.0048) centre (-149.5676, -111.6566) ccw projected
  arc A758 (-150.5836, -110.5312) -> (-150.9158, -111.1798) centre (-148.3337, -112.0931) ccw projected
  arc A759 (-150.5836, -110.5312) -> (-150.6627, -109.8326) centre (-151.0218, -110.2271) ccw projected
  arc A760 (-150.6627, -109.8326) -> (-151.2639, -109.2954) centre (-180.2765, -142.3655) ccw projected
  arc A761 (-151.2639, -109.2954) -> (-151.967, -109.295) centre (-151.6156, -109.6964) ccw projected
  arc A762 (-152.5742, -109.6977) -> (-151.967, -109.295) centre (-153.7709, -107.2342) ccw projected
  arc A763 (-154.5921, -108.0885) -> (-152.5742, -109.6977) centre (-153.199, -108.4114) ccw projected
  arc A764 (-154.3346, -107.4069) -> (-154.5921, -108.0885) centre (-151.924, -108.707) ccw projected
  arc A765 (-154.3346, -107.4069) -> (-154.4914, -106.7215) centre (-154.8041, -107.1537) ccw projected
  arc A766 (-154.4914, -106.7215) -> (-155.149, -106.2549) centre (-180.2765, -142.3655) ccw projected
  arc A767 (-155.149, -106.2549) -> (-155.8477, -106.3333) centre (-155.4536, -106.6928) ccw projected
  arc A768 (-156.406, -106.8014) -> (-155.8477, -106.3333) centre (-157.871, -104.4874) ccw projected
  arc A769 (-158.5914, -105.4283) -> (-156.406, -106.8014) centre (-157.1709, -105.5932) ccw projected
  arc A770 (-158.4118, -104.7221) -> (-158.5914, -105.4283) centre (-155.8709, -105.7441) ccw projected
  arc A771 (-158.4118, -104.7221) -> (-158.6444, -104.0586) centre (-158.9067, -104.5231) ccw projected
  arc A772 (-158.6444, -104.0586) -> (-159.3501, -103.6686) centre (-180.2765, -142.3655) ccw projected
  arc A773 (-159.3501, -103.6686) -> (-160.0356, -103.8247) centre (-159.6038, -104.1378) ccw projected
  arc A774 (-160.538, -104.3524) -> (-160.0356, -103.8247) centre (-162.2529, -102.2169) ccw projected
  arc A775 (-162.8634, -103.2326) -> (-160.538, -104.3524) centre (-161.4334, -103.2374) ccw projected
  arc A776 (-162.764, -102.5107) -> (-162.8634, -103.2326) centre (-160.1246, -103.2418) ccw projected
  arc A777 (-162.764, -102.5107) -> (-163.0695, -101.8774) centre (-163.2781, -102.3683) ccw projected
  arc A778 (-163.0695, -101.8774) -> (-163.8143, -101.5689) centre (-180.2765, -142.3655) ccw projected
  arc A779 (-163.8143, -101.5689) -> (-164.4781, -101.8007) centre (-164.0139, -102.0636) ccw projected
  arc A780 (-164.9183, -102.3814) -> (-164.4781, -101.8007) centre (-166.8614, -100.4513) ccw projected
  arc A781 (-167.3544, -101.529) -> (-164.9183, -102.3814) centre (-165.9328, -101.3737) ccw projected
  arc A782 (-167.3365, -100.8006) -> (-167.3544, -101.529) centre (-164.6318, -101.2315) ccw projected
  arc A783 (-167.3365, -100.8006) -> (-167.7109, -100.2054) centre (-167.8632, -100.7166) ccw projected
  arc A784 (-167.7109, -100.2054) -> (-168.4856, -99.9822) centre (-180.2765, -142.3655) ccw projected
  arc A785 (-168.4856, -99.9822) -> (-169.1192, -100.2869) centre (-168.6286, -100.4961) ccw projected
  arc A786 (-169.4916, -100.9133) -> (-169.1192, -100.2869) centre (-171.6387, -99.2129) ccw projected
  arc A787 (-172.0079, -100.3389) -> (-169.4916, -100.9133) centre (-170.6127, -100.0254) ccw projected
  arc A788 (-172.0716, -99.6131) -> (-172.0079, -100.3389) centre (-169.3357, -99.7385) ccw projected
  arc A789 (-172.0716, -99.6131) -> (-172.5103, -99.0636) centre (-172.6045, -99.5887) ccw projected
  arc A790 (-172.5103, -99.0636) -> (-173.3052, -98.9286) centre (-180.2765, -142.3655) ccw projected
  arc A791 (-173.3052, -98.9286) -> (-173.9007, -99.3023) centre (-173.3897, -99.4552) ccw projected
  arc A792 (-174.2006, -99.9664) -> (-173.9007, -99.3023) centre (-176.5245, -98.5171) ccw projected
  arc A793 (-176.7654, -99.6774) -> (-174.2006, -99.9664) centre (-175.414, -99.2097) ccw projected
  arc A794 (-176.91, -98.9632) -> (-176.7654, -99.6774) centre (-174.1772, -98.7816) ccw projected
  arc A795 (-176.91, -98.9632) -> (-177.4074, -98.4664) centre (-177.4422, -98.9986) ccw projected
  arc A796 (-177.4074, -98.4664) -> (-178.2124, -98.4212) centre (-180.2765, -142.3655) ccw projected
  arc A797 (-178.2124, -98.4212) -> (-178.7623, -98.8592) centre (-178.2374, -98.954) ccw projected
  arc A798 (-178.986, -99.5527) -> (-178.7623, -98.8592) centre (-181.4576, -98.3727) ccw projected
  arc A799 (-181.567, -99.5527) -> (-178.986, -99.5527) centre (-180.2765, -98.9366) ccw projected
  arc A800 (-181.7907, -98.8592) -> (-181.567, -99.5527) centre (-179.0954, -98.3727) ccw projected
  circle A801 centre (-171.542, -73.2557) radius 25.4
  line L47 (-171.542, -73.2557) -> (-105.9978, 19.434)
  line L48 (-171.542, -73.2557) -> (-150.8033, -87.9208)
  line L49 (-171.542, -73.2557) -> (-192.2807, -58.5906)
  line L50 (-171.6886, -73.4631) -> (-155.4522, -92.9961)
  line L51 (-171.6886, -73.4631) -> (-187.9251, -53.9301)
  line L52 (-171.8353, -73.6705) -> (-161.2076, -96.7402)
  line L53 (-171.8353, -73.6705) -> (-182.463, -50.6008)
  line L54 (-171.6886, -73.4631) -> (-152.6538, -57.6407)
  line L55 (-171.8353, -73.6705) -> (-149.3539, -63.3138)
  line L56 (-171.542, -73.2557) -> (-185.8331, -93.4656)
  line L57 (-171.6886, -73.4631) -> (-190.7235, -89.2855)
  line L58 (-171.8353, -73.6705) -> (-194.3167, -84.0272)
  circle A802 centre (-171.542, -73.2557) radius 24.7523
  point P0 (-157.2508, -53.0458)
  dimension "d876" = 113.5228
  dimension "d877" = 28.5496
  dimension "d878" = 27.94
  dimension "d879" = 42.9717
  dimension "d880" = 44.45
  dimension "d881" = 44.45
  dimension "d882" = 50.8
  dimension "d883" = 28.6487
  dimension "d886" = 0.254
  dimension "d891" = 15
  dimension "d892" = 15
  dimension "d893" = 15
  dimension "d894" = 15
  dimension "d927" = 49.5046
  constraints: 44 end point, 16 coincident, 8 equal length, 8 point on circle, 7 midpoint, 5 centre point, 5 collinear, 4 tangent, 3 perpendicular, 2 parallel, 1 horizontal, 1 point on line, 6 other
  measures "d876" distance of point (-105.998, 19.434) point (-171.542, -73.256)
  measures "d877" diameter of A457
  measures "d878" distance from line of point (-171.542, -73.256) L32
  measures "d879" diameter of A458
  measures "d880" distance of L43.end L41.start
  measures "d881" distance of L41.start L41.end
  measures "d882" diameter of A801
  measures "d883" diameter of A459
  measures "d886" distance of point (-171.542, -73.256) L50.start
  measures "d891" angle of L48 L50
  measures "d892" angle of L50 L52
  measures "d893" angle of L54 L47
  measures "d894" angle of L55 L54
  measures "d927" diameter of A802
hole "Hole15" at (0, -53.0458, 157.2508) at (0, -87.9208, 150.8033) at (0, -58.5906, 192.2807) at (0, -92.9961, 155.4522) at (0, -53.9301, 187.9251) at (0, -50.6008, 182.463) at (0, -96.7402, 161.2076) at (0, -57.6407, 152.6538) at (0, -63.3138, 149.3539) at (0, -93.4656, 185.8331) at (0, -89.2855, 190.7235) at (0, -84.0272, 194.3167) direction (-1, 0, 0) diameter 4.318 end through all clearance for "Flat Head Machine Screw (82)" size "#8" standard "Ansi Unified Screw Threads"